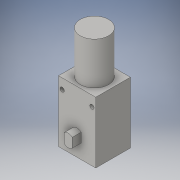
# Autodesk Inventor part: msheehan_motor
Saved by Autodesk Inventor 2016 (Build 200138000, 138)
## iProperties
Created: 2017-08-30
Part Number: msheehan_motor
Material: Generic
Document SubType Name: Modeling
Designer: student
Density: 1 g/cm^3
Appearance: Default
Author: student
Autodesk Inventor part; units mm, degrees
ref_plane "YZ Plane" through (0, 0, 0) normal (1, 0, 0) x (0, 1, 0)
ref_plane "XZ Plane" through (0, 0, 0) normal (0, 1, 0) x (-1, 0, 0)
ref_plane "XY Plane" through (0, 0, 0) normal (0, 0, 1) x (1, 0, 0)
sketch "Sketch1" plane through (0, 0, 0) normal (0, 0, 1) x (1, 0, 0)
  line L0 (0, 0) -> (22.352, 0)
  line L1 (22.352, 0) -> (22.352, 36.83)
  line L2 (22.352, 36.83) -> (0, 36.83)
  line L3 (0, 36.83) -> (0, 0)
  dimension "d0" = 22.352
  dimension "d1" = 36.83
  constraints: 8 end point, 2 parallel, 1 horizontal, 1 perpendicular
  measures "d0" distance of L2.end L1.end
  measures "d1" distance of L1.end L0.end
extrude "Extrusion1" add sketch "Sketch1" along normal blind 20.828
sketch "Sketch2" plane through (0, 36.83, 0) normal (0, 1, 0) x (1, 0, 0)
  circle A0 centre (11.176, -10.414) radius 8.509
  point P0 (0, 0)
  dimension "d4" = 17.018
  constraints: 1 centre point
  measures "d4" diameter of A0
extrude "Extrusion2" add sketch "Sketch2" along normal blind 25.4
sketch "Sketch3" plane through (0, 0, 0) normal (0, 0, -1) x (-1, 0, 0)
  point P0 (0, 0)
sketch "Sketch4" plane through (0, 0, 20.828) normal (0, 0, 1) x (1, 0, 0)
  line L0 (22.352, 36.83) -> (0, 36.83) projected
  line L1 (0, 36.83) -> (0, 0) projected
  circle A0 centre (2.2352, 30.734) radius 1.27
  line L2 (22.352, 0) -> (22.352, 36.83) projected
  circle A1 centre (20.1168, 30.734) radius 1.27
  dimension "d9" = 2.54
  dimension "d12" = 2.54
  constraints: 2 centre point
  measures "d9" diameter of A0
  measures "d12" diameter of A1
extrude "Extrusion3" cut sketch "Sketch4" against normal blind 25.4
sketch "Sketch5" plane through (0, 0, 0) normal (0, 0, -1) x (-1, 0, 0)
  point P0 (0, 0)
sketch "Sketch6" plane through (0, 0, 20.828) normal (0, 0, 1) x (1, 0, 0)
  line L0 (0, 0) -> (22.352, 0) projected
  line L1 (11.176, 0) -> (11.176, 7.62)
  line L2 (22.352, 0) -> (22.352, 11.43)
  line L3 (22.352, 11.43) -> (13.589, 11.43)
  line L4 (0, 11.43) -> (8.763, 11.43)
  line L5 (13.589, 8.5992) -> (13.589, 14.2608)
  line L6 (8.763, 14.3275) -> (8.763, 8.5325)
  line L7 (8.763, 7.6515) -> (13.589, 15.2085) construction
  line L8 (13.589, 7.6515) -> (8.763, 15.2085) construction
  arc A0 (8.763, 8.5325) -> (13.589, 8.5992) centre (11.14, 11.1716) ccw
  arc A1 (13.589, 14.2608) -> (8.763, 14.3275) centre (11.14, 11.6884) ccw
  point P0 (11.176, 11.43)
  dimension "d16" = 7.62
  dimension "d17" = 11.43
  dimension "d18" = 8.763
  constraints: 16 end point, 5 point on circle, 5 symmetric about line, 3 midpoint, 2 centre point, 2 vertical, 1 parallel, 1 perpendicular, 1 other
  measures "d16" distance of L1.start L1.end
  measures "d17" distance of L0.end L2.end
  measures "d18" distance of L2.end L3.end
extrude "Extrusion4" add sketch "Sketch6" along normal blind 5.334 contours A0 L6 A1 L5
body "Solid1"
